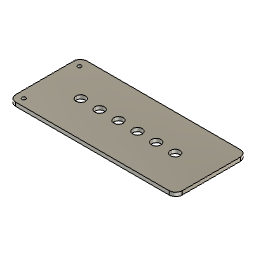
JM_pickup_v2 (Autodesk Fusion 360 design; units mm, degrees)
Autodesk Fusion 360 part; units mm, degrees
sketch "スケッチ1" plane through (0, 0, 0) normal (0, 0, 1) x (1, 0, 0)
  line L0 (3.5, 0) -> (86.5, 0)
  line L1 (90, 3.5) -> (90, 35)
  line L2 (86.5, 38.5) -> (3.5, 38.5)
  line L3 (0, 35) -> (0, 3.5)
  line L4 (0, 19.25) -> (90, 19.25)
  arc A0 (3.5, 38.5) -> (0, 35) centre (3.5, 35) ccw
  arc A1 (90, 35) -> (86.5, 38.5) centre (86.5, 35) ccw
  arc A2 (86.5, 0) -> (90, 3.5) centre (86.5, 3.5) ccw
  arc A3 (0, 3.5) -> (3.5, 0) centre (3.5, 3.5) ccw
  point P0 (90, 0)
  point P1 (0, 38.5)
  dimension "d1" = 90
  dimension "d2" = 38.5
  dimension "d3" = 3.5
  constraint horizontal L0
  constraint vertical L1
  constraint horizontal L2
  constraint vertical L3
  constraint coincident L3 L4.start
  constraint coincident P1 L2
  constraint coincident P1 L3
  constraint tangent L2 A0
  constraint tangent L3 A0
  constraint coincident L1 L4.end
  constraint tangent L1 A1
  constraint tangent L2 A1
  constraint equal A0 A1
  constraint coincident P0 L0
  constraint coincident P0 L1
  constraint tangent L0 A2
  constraint tangent L1 A2
  constraint equal A0 A2
  constraint coincident origin L0
  constraint coincident origin L3
  constraint tangent L0 A3
  constraint tangent L3 A3
  constraint equal A0 A3
  measures "d1" distance of origin P0
  measures "d2" distance of origin P1
  measures "d3" radius of A0
extrude "押し出し1" add sketch "スケッチ1" along normal blind 2
sketch "スケッチ2" plane through (0, 0, 2) normal (0, 0, 1) x (-1, 0, 0)
  arc A0 (0, -3.5) -> (-3.5, 0) centre (-3.5, -3.5) ccw
  line L0 (-3.5, 0) -> (-86.5, 0)
  arc A1 (-86.5, 0) -> (-90, -3.5) centre (-86.5, -3.5) ccw
  line L1 (-90, -3.5) -> (-90, -35)
  arc A2 (-90, -35) -> (-86.5, -38.5) centre (-86.5, -35) ccw
  line L2 (-86.5, -38.5) -> (-3.5, -38.5)
  arc A3 (-3.5, -38.5) -> (0, -35) centre (-3.5, -35) ccw
  line L3 (0, -35) -> (0, -3.5)
  line L4 (-45, -38.5) -> (-45, 0)
  line L5 (0, -19.25) -> (-90, -19.25)
  line L6 (-45, -19.25) -> (-50.1, -19.25)
  line L7 (-50.1, -19.25) -> (-60.3, -19.25)
  line L8 (-60.3, -19.25) -> (-70.5, -19.25)
  point P0 (-50.1, -19.25)
  point P1 (-60.3, -19.25)
  point P2 (-70.5, -19.25)
  point P3 (-39.9, -19.25)
  point P4 (-29.7, -19.25)
  point P5 (-19.5, -19.25)
  dimension "d6" = 5.1
  dimension "d7" = 10.2
  dimension "d8" = 10.2
  constraint midpoint L2 L4.start
  constraint midpoint L0 L4.end
  constraint midpoint L3 L5.start
  constraint midpoint L1 L5.end
  constraint midpoint L4 L6.start
  constraint perpendicular L4 L6
  constraint coincident P0 L6.end
  constraint parallel L5 L7
  constraint coincident P1 L7.end
  constraint coincident L5 P2
  constraint coincident P2 L8.end
  constraint symmetric L4 P0 P3
  constraint symmetric L4 P1 P4
  constraint symmetric L4 P2 P5
  measures "d6" distance of L6.start P0
  measures "d7" distance of P0 P1
  measures "d8" distance of P1 P2
hole "穴1" at (19.5, 19.25, 2) at (29.7, 19.25, 2) at (39.9, 19.25, 2) at (50.1, 19.25, 2) at (60.3, 19.25, 2) at (70.5, 19.25, 2) direction (0, 0, -1) diameter 5.1 depth 2 tip angle 180
sketch "スケッチ3" plane through (0, 0, 2) normal (0, 0, 1) x (-1, 0, 0)
  circle A0 centre (-60.3, -19.25) radius 2.55
  circle A1 centre (-39.9, -19.25) radius 2.55
  circle A2 centre (-19.5, -19.25) radius 2.55
  circle A3 centre (-29.7, -19.25) radius 2.55
  circle A4 centre (-50.1, -19.25) radius 2.55
  circle A5 centre (-70.5, -19.25) radius 2.55
  arc A6 (0, -3.5) -> (-3.5, 0) centre (-3.5, -3.5) ccw
  line L0 (-3.5, 0) -> (-86.5, 0)
  arc A7 (-86.5, 0) -> (-90, -3.5) centre (-86.5, -3.5) ccw
  line L1 (-90, -3.5) -> (-90, -35)
  arc A8 (-90, -35) -> (-86.5, -38.5) centre (-86.5, -35) ccw
  line L2 (-86.5, -38.5) -> (-3.5, -38.5)
  arc A9 (-3.5, -38.5) -> (0, -35) centre (-3.5, -35) ccw
  line L3 (0, -35) -> (0, -3.5)
  line L4 (-4, -4) -> (-4, -34)
  constraint perpendicular L0 L4
hole "穴2" at (4, 4, 2) at (4, 34, 2) direction (0, 0, -1) diameter 2 depth 2 tip angle 180
sketch "スケッチ5" plane through (0, 0, 0) normal (0, 0, 1) x (1, 0, 0)
sketch "スケッチ6" plane through (0, 0, 0) normal (0, 0, 1) x (1, 0, 0)
